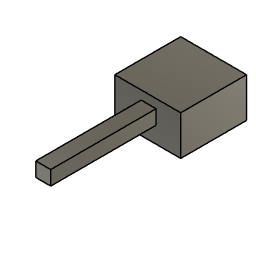
Cantilever Structural analysis (Autodesk Fusion 360 design; units mm, degrees)
Autodesk Fusion 360 part; units mm, degrees
sketch "Sketch1" plane through (0, 0, 0) normal (0, 0, 1) x (1, 0, 0)
  line L0 (-50, 65) -> (25, 65)
  line L1 (25, 65) -> (25, -10)
  line L2 (25, -10) -> (-50, -10)
  line L3 (-50, -10) -> (-50, 65)
  constraint horizontal L0
  constraint vertical L1
  constraint horizontal L2
  constraint vertical L3
extrude "Extrude1" add sketch "Sketch1" along normal blind 45
sketch "Sketch2" plane through (0, -10, 0) normal (0, -1, 0) x (1, 0, 0)
  line L0 (-50, 0) -> (25, 0)
  line L1 (25, 0) -> (25, 45)
  line L2 (25, 45) -> (-50, 45)
  line L3 (-50, 45) -> (-50, 0)
  line L4 (-20, 35) -> (-2.9952, 35)
  line L5 (-2.9952, 35) -> (-2.9952, 18.7359)
  line L6 (-2.9952, 18.7359) -> (-20, 18.7359)
  line L7 (-20, 18.7359) -> (-20, 35)
  constraint horizontal L4
  constraint vertical L5
  constraint horizontal L6
  constraint vertical L7
extrude "Extrude2" add sketch "Sketch2" along normal blind 120 contours L4 L5 L6 L7
